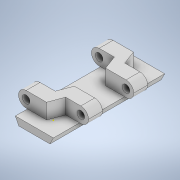
# Autodesk Inventor part: pás-tiger I
Saved by Autodesk Inventor 2022 (Build 260153000, 153)
## iProperties
Created: 2022-10-30
Part Number: pás-tiger I
Material: Generic
Document SubType Name: Modeling
Designer: matys
Density: 1 g/cm^3
Appearance: Default
Author: matys
Autodesk Inventor part; units mm, degrees
ref_plane "YZ Plane" through (0, 0, 0) normal (1, 0, 0) x (0, 1, 0)
ref_plane "XZ Plane" through (0, 0, 0) normal (0, 1, 0) x (-1, 0, 0)
ref_plane "XY Plane" through (0, 0, 0) normal (0, 0, 1) x (1, 0, 0)
sketch "Sketch1" plane through (0, 0, 0) normal (0, 1, 0) x (-1, 0, 0)
  line L0 (0, 0) -> (0, -32)
  line L1 (0, -32) -> (10.9556, -32)
  line L2 (10.9556, -32) -> (10.9556, 0)
  line L3 (10.9556, 0) -> (0, 0)
  dimension "d0" = 32
  dimension "d1" = 10.9556
  constraints: 8 end point, 2 perpendicular, 1 horizontal, 1 vertical
  measures "d0" distance of L0.start L0.end
  measures "d1" distance of L0.end L1.end
extrude "Extrusion1" add sketch "Sketch1" along normal blind 2
sketch "Sketch2" plane through (-10.9556, 0, 0) normal (0, 0, 1) x (1, 0, 0)
  line L0 (10.9556, 0) -> (0, 0) projected
  line L1 (10.9556, 0) -> (9.9556, 0)
  line L2 (9.9556, 0) -> (9.9556, 2)
  line L3 (10.9556, 2) -> (0, 2) projected
  line L4 (10.9556, 2) -> (9.9556, 0)
  line L5 (0, 0) -> (0, 2) projected
  line L6 (0, 0) -> (1, 0)
  line L7 (1, 0) -> (0, 2)
  line L8 (1, 0) -> (0, 0)
  line L9 (0, 2) -> (0, 0)
  line L10 (0, 2) -> (10.9556, 2)
  line L11 (9.9556, 0) -> (1, 0)
  line L12 (9.9556, 0) -> (10.9556, 0)
  line L13 (10.9556, 0) -> (10.9556, 2) projected
  line L14 (10.9556, 2) -> (10.9556, 0)
  line L15 (10.9556, 0) -> (9.9556, 0)
  dimension "d4" = 1
  dimension "d5" = 1
  constraints: 24 end point, 4 collinear, 3 point on line, 2 horizontal, 2 perpendicular
  measures "d4" distance of L0.start L1.end
  measures "d5" distance of L0.end L6.end
extrude "Extrusion2" cut sketch "Sketch2" against normal through all contours L0 L4 L13 | L0 L5 L7
sketch "Sketch3" plane through (0, 2, 0) normal (0, 1, 0) x (1, 0, 0)
  line L0 (-10.9556, 32) -> (-10.9556, 0) projected
  line L1 (-10.9556, 32) -> (-10.9556, 0)
  line L2 (-10.9556, 0) -> (-10.9556, 16)
  line L3 (-10.9556, 16) -> (0, 16)
  line L4 (0, 0) -> (0, 32) projected
  line L5 (-10.9556, 0) -> (0, 0) projected
  line L6 (0, 32) -> (-10.9556, 32) projected
  line L7 (-10.9556, 32) -> (-10.9556, 30)
  line L8 (-10.9556, 28.5) -> (0, 28.5)
  line L9 (-10.9556, 0) -> (-10.9556, 2)
  line L10 (-10.9556, 3.5) -> (0, 3.5)
  line L11 (-10.9556, 30) -> (-10.9556, 22)
  line L12 (-10.9556, 20.5) -> (0, 20.5)
  line L13 (-10.9556, 2) -> (-10.9556, 10)
  line L14 (-10.9556, 11.5) -> (0, 11.5)
  line L15 (-10.9556, 20.5) -> (-11.494, 20.5)
  line L16 (-11.494, 20.5) -> (-11.494, 28.5)
  line L17 (-11.494, 28.5) -> (-10.9556, 28.5)
  line L18 (-11.494, 28.5) -> (-13.5464, 28.5)
  line L19 (-13.5464, 28.5) -> (-13.5464, 20.5)
  line L20 (-13.5464, 20.5) -> (-11.494, 20.5)
  line L21 (-11.494, 28.5) -> (-12.994, 28.5)
  line L22 (-11.494, 28.5) -> (-9.994, 28.5)
  line L23 (0, 30) -> (0, 22)
  line L24 (0, 20.5) -> (0.538, 20.5)
  line L25 (0.538, 20.5) -> (0.538, 28.5)
  line L26 (0.538, 28.5) -> (0, 28.5)
  line L27 (0.538, 28.5) -> (2.59, 28.5)
  line L28 (2.59, 28.5) -> (2.59, 20.5)
  line L29 (2.59, 20.5) -> (0.538, 20.5)
  line L30 (0.538, 28.5) -> (2.038, 28.5)
  line L31 (2.038, 28.5) -> (2.038, 20.5)
  line L32 (0.538, 28.5) -> (-0.962, 28.5)
  line L33 (-0.962, 30) -> (-0.962, 22)
  line L34 (-10.9556, 11.5) -> (-11.4936, 11.5)
  line L35 (-11.4936, 11.5) -> (-13.5456, 11.5)
  line L36 (-13.5456, 11.5) -> (-13.5456, 3.5)
  line L37 (-13.5456, 3.5) -> (-10.9556, 3.5)
  line L38 (0, 11.5) -> (0.538, 11.5)
  line L39 (0.538, 11.5) -> (2.59, 11.5)
  line L40 (2.59, 11.5) -> (2.59, 3.5)
  line L41 (2.59, 3.5) -> (0, 3.5)
  line L42 (0, 10) -> (0, 11.5)
  line L43 (0, 11.5) -> (-10.9556, 11.5)
  line L44 (0, 22) -> (0, 20.5)
  dimension "d8" = 32
  dimension "d10" = 2
  dimension "d11" = 2
  dimension "d12" = 8
  dimension "d13" = 8
  dimension "d14" = 0.5384
  dimension "d15" = 2.0524
  dimension "d16" = 1.5
  dimension "d17" = 1.5
  dimension "d23" = 0.538
  dimension "d24" = 2.052
  dimension "d25" = 1.5
  dimension "d26" = 1.5
  dimension "d27" = 0.538
  dimension "d28" = 2.052
  dimension "d29" = 0.538
  dimension "d43" = 1.5
  dimension "d44" = 1.5
  constraints: 82 end point, 19 perpendicular, 11 point on line, 3 horizontal, 2 collinear, 2 midpoint, 1 parallel
  measures "d8" distance of L0.start L0.end
  measures "d10" distance of L7.end L0.start
  measures "d11" distance of L9.end L0.end
  measures "d12" distance of L11.start L11.end
  measures "d13" distance of L13.start L13.end
  measures "d14" distance of L12.start L15.end
  measures "d15" distance of L17.start L18.end
  measures "d16" distance of L17.start L21.end
  measures "d17" distance of L17.start L22.end
  measures "d23" distance of L24.start L24.end
  measures "d24" distance of L25.end L27.end
  measures "d25" distance of L25.end L30.end
  measures "d26" distance of L25.end L32.end
  measures "d27" distance of L14.start L34.end
  measures "d28" distance of L34.end L35.end
  measures "d29" distance of L38.start L38.end
  measures "d43" distance of L42.start L42.end
  measures "d44" distance of L44.start L44.end
extrude "Extrusion3" add sketch "Sketch3" along normal blind 4.4114 contours L8 L4 L12 L0 | L0 L15 L16 L17 | L16 L20 L19 L18 | L26 L25 L24 L4 | L27 L31 L29 L25 | L27 L28 L29 L31 | L14 L4 L10 L0 | L0 L37 L36 L35 L34 | L38 L39 L40 L41 L4
fillet "Fillet1" radius 2.2055 8 edges at (2.59, 6.4114, -7.5) (2.59, 2, -7.5) (2.59, 6.4114, -24.5) (2.59, 2, -24.5) (-13.5464, 6.4114, -24.5) (-13.5464, 2, -24.5) (-13.5456, 6.4114, -7.5) (-13.5456, 2, -7.5)
sketch "Sketch4" plane through (0, 6.4114, 0) normal (0, 1, 0) x (1, 0, 0)
  line L0 (-11.3401, 3.5) -> (-11.3401, 11.5) projected
  line L1 (-11.3401, 11.5) -> (-11.3401, 3.5)
  line L2 (-11.3401, 3.5) -> (-11.3401, 7.5)
  line L3 (-11.3401, 7.5) -> (-13.5456, 7.5)
  line L4 (-13.5456, 3.5) -> (-13.5456, 11.5) projected
  line L5 (-11.3401, 7.5) -> (2.59, 7.5)
  line L6 (2.59, 11.5) -> (2.59, 3.5) projected
  line L7 (0.3845, 3.5) -> (0.3845, 11.5) projected
  line L8 (-10.9556, 11.5) -> (0, 11.5) projected
  line L9 (-5.4778, 11.5) -> (-5.4778, 3.5)
  line L10 (-11.3401, 3.5) -> (0.3845, 3.5) projected
  line L11 (-5.4778, 7.5) -> (-6.9778, 7.5)
  line L12 (-6.9778, 7.5) -> (-5.4778, 11.5)
  line L13 (-5.4778, 7.5) -> (-3.9778, 7.5)
  line L14 (-3.9778, 7.5) -> (-5.4778, 3.5)
  line L15 (2.59, 2) -> (0.3845, 2) projected
  line L16 (-5.4778, 3.5) -> (2.59, 3.5)
  line L17 (2.59, 3.5) -> (2.59, 7.5)
  line L18 (-13.5456, 7.5) -> (-13.5456, 11.5)
  line L19 (-13.5456, 11.5) -> (-11.3401, 11.5) projected
  line L20 (-5.4778, 11.5) -> (-13.5456, 11.5)
  line L21 (-13.5456, 11.5) -> (-13.5456, 7.5)
  line L22 (-11.3409, 28.5) -> (-11.3409, 20.5) projected
  line L23 (-11.3409, 28.5) -> (-11.3409, 20.5)
  line L24 (-11.3409, 20.5) -> (-11.3409, 24.5)
  line L25 (-11.3409, 24.5) -> (0.3845, 24.5)
  line L26 (0.3845, 24.5) -> (-5.4782, 24.5)
  line L27 (-5.4782, 28.5) -> (-5.4782, 24.5)
  line L28 (-5.4782, 24.5) -> (-5.4782, 20.5)
  line L29 (-5.4782, 20.5) -> (-5.4782, 24.5)
  line L30 (-5.4782, 24.5) -> (-3.9782, 24.5)
  line L31 (-3.9782, 24.5) -> (-5.4782, 28.5)
  line L32 (-5.4782, 24.5) -> (-6.9782, 24.5)
  line L33 (-6.9782, 24.5) -> (-5.4782, 20.5)
  line L34 (-13.5464, 20.5) -> (-13.5464, 28.5) projected
  line L35 (-5.4782, 20.5) -> (-13.5464, 20.5)
  line L36 (-13.5464, 20.5) -> (-13.5464, 24.5)
  line L37 (-13.5464, 24.5) -> (-6.9782, 24.5)
  line L38 (-10.9556, 28.5) -> (0, 28.5) projected
  line L39 (-3.9782, 24.5) -> (4.3111, 24.5)
  line L40 (4.3111, 24.5) -> (4.3111, 28.5)
  line L41 (-5.4782, 28.5) -> (4.3111, 28.5)
  line L42 (0.3845, 28.5) -> (-11.3409, 28.5) projected
  point P0 (0, 0)
  point P1 (2.59, 10)
  point P2 (0.3845, 10)
  point P3 (0, 10)
  point P4 (0, 28.5)
  point P5 (-3.9782, 24.5)
  dimension "d33" = 1.5
  dimension "d34" = 1.5
  dimension "d37" = 1.5
  dimension "d38" = 1.5
  constraints: 62 end point, 8 midpoint, 7 point on line, 6 collinear, 3 horizontal, 3 perpendicular, 2 parallel, 1 vertical, 2 other
  measures "d33" distance of L11.start L11.end
  measures "d34" distance of L11.start L13.end
  measures "d37" distance of L26.end L30.end
  measures "d38" distance of L26.end L32.end
extrude "Extrusion4" cut sketch "Sketch4" against normal blind 4.4114 contours L3 L4 L19 L0 | L0 L20 L8 L12 L5 | L14 L5 L7 L10 | L7 L5 L6 L16 | L25 L33 L35 L22 | L22 L35 L34 L37 | L38 L41 L40 L39 L25 L31
sketch "Sketch5" plane through (-3.9778, 6.4114, -7.5) normal (0, 0, 1) x (1, 0, 0)
  arc A0 (6.5678, -2.2055) -> (4.3623, 0) centre (4.3623, -2.2055) ccw projected
  line L0 (4.3623, 0) -> (4.3623, -2.2055)
  arc A1 (-7.3631, 0) -> (-9.5686, -2.2055) centre (-7.3631, -2.2055) ccw projected
  line L1 (-7.3631, 0) -> (-7.3631, -2.2055)
  circle A2 centre (-7.3631, -2.2055) radius 1.1
  circle A3 centre (4.3623, -2.2055) radius 1.1
  point P0 (3.9778, -6.4114)
  dimension "d39" = 2.2
  dimension "d40" = 2.2
  constraints: 4 end point, 2 centre point, 2 coincident, 2 vertical, 1 point on circle
  measures "d39" diameter of A2
  measures "d40" diameter of A3
extrude "Extrusion5" cut sketch "Sketch5" along normal through all both and the other way through all
sketch "Sketch6" plane through (0, 6.4114, 0) normal (0, 1, 0) x (1, 0, 0)
  point P0 (0, 0)
body "Solid1"
